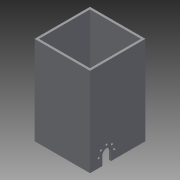
# Autodesk Inventor part: Arm_Fifth_Flame
Saved by Autodesk Inventor 2013 (Build 170138000, 138)
## iProperties
Created: 2014-04-18
Part Number: Arm_Fifth_Flame
Material: 一般
Document SubType Name: Modeling
Designer: andou
Density: 1 g/cm^3
Author: andou
Autodesk Inventor part; units mm, degrees
ref_plane "YZ Plane" through (0, 0, 0) normal (1, 0, 0) x (0, 1, 0)
ref_plane "XZ Plane" through (0, 0, 0) normal (0, 1, 0) x (-1, 0, 0)
ref_plane "XY Plane" through (0, 0, 0) normal (0, 0, 1) x (1, 0, 0)
sketch "スケッチ1" plane through (0, 0, 0) normal (0, 0, 1) x (1, 0, 0)
  line L0 (-25, 25) -> (25, 25)
  line L1 (25, 25) -> (25, -25)
  line L2 (25, -25) -> (-25, -25)
  line L3 (-25, -25) -> (-25, 25)
  line L4 (-23, 23) -> (23, 23)
  line L5 (23, 23) -> (23, -23)
  line L6 (23, -23) -> (-23, -23)
  line L7 (-23, -23) -> (-23, 23)
  point P0 (0, 0)
  dimension "d0" = 50
  dimension "d2" = 50
  dimension "d3" = 46
  dimension "d4" = 23
  dimension "d5" = 23
  dimension "d6" = 25
  dimension "d7" = 46
  dimension "d8" = 25
  constraints: 16 end point, 4 parallel, 2 horizontal, 2 perpendicular
  measures "d0" distance of L0.start L0.end
  measures "d2" distance of L2.end L0.start
  measures "d3" distance of L5.end L6.end
  measures "d4" distance from line of point (0, 0) L7
  measures "d5" distance from line of point (0, 0) L6
  measures "d6" distance from line of point (0, 0) L0
  measures "d7" distance between parallel lines of L6 L4
  measures "d8" distance from line of L1 point (0, 0)
extrude "押し出し1" add sketch "スケッチ1" against normal blind 80
sketch "スケッチ2" plane through (25, -25, 0) normal (1, 0, 0) x (0, 0, -1)
  line L0 (0, 0) -> (80, 0) projected
  line L1 (80, 50) -> (80, 0) projected
  line L2 (80, 19) -> (72, 19)
  line L3 (72, 11) -> (80, 11)
  line L4 (80, 11) -> (80, 19)
  arc A0 (72, 19) -> (72, 11) centre (72, 15) ccw
  point P0 (0, 25)
  dimension "d11" = 8
  dimension "d15" = 4
  dimension "d16" = 8
  dimension "d17" = 15
  dimension "d18" = 8
  dimension "d19" = 8
  constraints: 6 end point, 2 point on circle, 1 centre point, 1 horizontal, 1 parallel, 1 point on line
  measures "d11" distance between parallel lines of L3 L2
  measures "d15" radius of A0
  measures "d16" distance from line of L1 A0.centre
  measures "d17" distance from line of L0 A0.centre
  measures "d18" distance of L3.start L3.end
  measures "d19" distance of L2.start L2.end
extrude "押し出し2" cut sketch "スケッチ2" against normal blind 60
sketch "スケッチ3" plane through (25, -25, 0) normal (1, 0, 0) x (0, 0, -1)
  arc A0 (72, 19) -> (72, 11) centre (72, 15) ccw projected
  circle A1 centre (72, 22) radius 1
  point P0 (0, 25)
  dimension "d22" = 0
  dimension "d23" = 7
  dimension "d24" = 2
  constraints: 1 centre point
  measures "d22" horizontal distance of A1.centre A0.centre
  measures "d23" distance of A1.centre A0.centre
  measures "d24" diameter of A1
hole "穴1" at (25, -3, -72) direction (-1, 0, 0) diameter 2 end through all
pattern_circular "円形状パターン1" count 5 over 180 about axis through (25, -10, -72) along (1, 0, 0) of "穴1"
sketch "スケッチ4" plane through (-25, 25, 0) normal (0, 1, 0) x (1, 0, 0)
  line L0 (50, 0) -> (50, 80) projected
  line L1 (0, 80) -> (50, 80) projected
  line L2 (2, 80) -> (48, 80)
  line L3 (48, 80) -> (48, 45)
  line L4 (48, 45) -> (2, 45)
  line L5 (2, 45) -> (2, 80)
  point P0 (25, 0)
  dimension "d35" = 46
  dimension "d37" = 2
  dimension "d38" = 35
  constraints: 8 end point, 2 parallel, 1 horizontal, 1 perpendicular, 1 point on line
  measures "d35" distance of L3.end L4.end
  measures "d37" distance between parallel lines of L0 L3
  measures "d38" distance between parallel lines of L1 L4
extrude "押し出し3" cut sketch "スケッチ4" against normal blind 30
